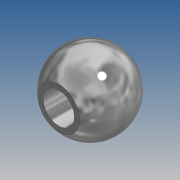
# Autodesk Inventor part: Boule_Rotule_M2
Saved by Autodesk Inventor 2021.3 (Build 253353000, 353)
## iProperties
Created: 2023-08-17
Part Number: Boule_Rotule_M2
Material: C45E (Ck45)
Document SubType Name: Modeling
Designer: cedric.clivaz
Density: 7.85 g/cm^3
Appearance: Polished - Small Pyramid Knurl
Author: cedric.clivaz
Autodesk Inventor part; units mm, degrees
ref_plane "YZ Plane" through (0, 0, 0) normal (1, 0, 0) x (0, 1, 0)
ref_plane "XZ Plane" through (0, 0, 0) normal (0, 1, 0) x (-1, 0, 0)
ref_plane "XY Plane" through (0, 0, 0) normal (0, 0, 1) x (1, 0, 0)
sketch "Sketch2" plane through (0, 0, 0) normal (0, 0, 1) x (1, 0, 0)
  line L0 (-3.36, 0) -> (3.36, 0) construction
  arc A0 (2.4, 0) -> (-2.4, 0) centre (0, 0) ccw
  line L1 (-2.4, 0) -> (2.4, 0)
  dimension "d0" = 4.8
  constraints: 2 end point, 2 point on circle, 2 point on line, 1 centre point, 1 coincident
  measures "d0" diameter of A0
revolve "Revolution1" add sketch "Sketch2" angle 360 about axis through (-10, 0, 0) along (1, 0, 0)
sketch "Sketch3" plane through (0, 0, 0) normal (0, 1, 0) x (-1, 0, 0)
  circle A0 centre (0, 0) radius 1
  dimension "d2" = 2
  constraints: 1 centre point, 1 coincident
  measures "d2" diameter of A0
extrude "Extrusion1" cut sketch "Sketch3" along normal through all both and the other way through all
sketch "Sketch4" plane through (0, 0, 0) normal (1, 0, 0) x (0, 1, 0)
  line L0 (2.1817, 1) -> (2.1817, -1) construction
  line L1 (-2.1817, -1) -> (-2.1817, 1) construction
  line L2 (0, -3.36) -> (0, 3.36) construction
  arc A0 (-2.1817, -1) -> (-2.1817, 1) centre (0, 0) ccw construction
  circle A1 centre (0, 0) radius 2.4
  line L3 (2, 1.3266) -> (2, -1.3266)
  line L4 (-2, 1.3266) -> (-2, -1.3266)
  dimension "d5" = 2
  dimension "d6" = 2
  constraints: 4 end point, 4 point on circle, 2 vertical, 1 centre point, 1 coincident, 1 concentric
  measures "d5" distance between parallel lines of L2 L3
  measures "d6" distance between parallel lines of L4 L2
extrude "Extrusion2" cut sketch "Sketch4" against normal through all both and the other way through all contours A1 L3 | L4 A1
equation "\"d6\" = d5"
body "Solid1"
